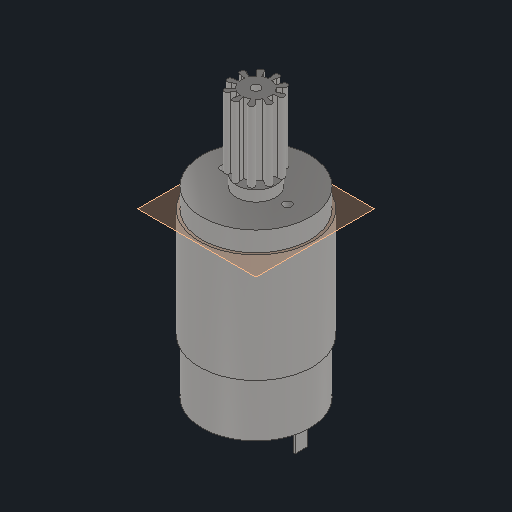
# Autodesk Inventor part: rs390
Saved by Autodesk Inventor 2023 (Build 270158000, 158)
## iProperties
Created: 2024-04-13
Part Number: rs390
Material: Steel, Mild
Document SubType Name: Modeling
Designer: szymo
Density: 7.85 g/cm^3
Appearance: Semi-Polished
Mass: 105 g
Surface Area: 71.7705 cm^2
Volume: 30.7913 cm^3
Author: szymo
Autodesk Inventor part; units mm, degrees
ref_plane "YZ Plane" through (0, 0, 0) normal (1, 0, 0) x (0, 1, 0)
ref_plane "XZ Plane" through (0, 0, 0) normal (0, 1, 0) x (-1, 0, 0)
ref_plane "XY Plane" through (0, 0, 0) normal (0, 0, 1) x (1, 0, 0)
sketch "Sketch1" plane through (0, 0, 0) normal (0, 1, 0) x (-1, 0, 0)
  circle A0 centre (0, 0) radius 13.7
  dimension "d0" = 27.4
  constraints: 1 centre point, 1 coincident
  measures "d0" diameter of A0
extrude "Extrusion1" add sketch "Sketch1" along normal blind 46.5
sketch "Sketch2" plane through (0, 46.5, 0) normal (0, 1, 0) x (1, 0, 0)
  circle A0 centre (0, 0) radius 13.7 projected
  circle A1 centre (0, 0) radius 5
  dimension "d3" = 10
  constraints: 1 centre point, 1 coincident
  measures "d3" diameter of A1
extrude "Extrusion2" add sketch "Sketch2" along normal blind 2.7 contours A1
sketch "Sketch3" plane through (0, 46.5, 0) normal (0, 1, 0) x (1, 0, 0)
  circle A0 centre (0, 0) radius 5 projected
  circle A1 centre (0, 0) radius 5 projected
  circle A2 centre (0, 0) radius 13.7 projected
  circle A3 centre (0, 0) radius 13.7 projected
  line L0 (-13.7, 0) -> (13.7, 0)
  point P0 (-8, 0)
  point P1 (8, 0)
  dimension "d6" = 16
  dimension "d7" = 5.7
  dimension "d8" = 5.7
  constraints: 2 end point, 2 point on circle, 2 point on line, 1 horizontal
  measures "d6" distance of point (-8, 0) point (8, 0)
  measures "d7" distance of L0.start point (-8, 0)
  measures "d8" distance of L0.end point (8, 0)
hole "Hole1" at (-8, 46.5, 0) at (8, 46.5, 0) direction (0, -1, 0) diameter 2.1129 depth 2.8 thread size "M2.6x0.45" class "6H" standard "ISO Metric profile"
ref_plane "Work Plane1" through (0, 41.5, 0) normal (0, 1, 0) x (1, 0, 0)
sketch "Sketch4" plane through (0, 41.5, 0) normal (0, 1, 0) x (1, 0, 0)
  circle A0 centre (0, 0) radius 14.375
  dimension "d17" = 28.75
  constraints: 1 centre point, 1 coincident
  measures "d17" diameter of A0
extrude "Extrusion3" add sketch "Sketch4" against normal blind 27.7
sketch "Sketch5" plane through (0, 0, 0) normal (0, -1, 0) x (1, 0, 0)
  circle A0 centre (0, 0) radius 5
  dimension "d20" = 10
  constraints: 1 centre point, 1 coincident
  measures "d20" diameter of A0
extrude "Extrusion4" add sketch "Sketch5" along normal blind 4
sketch "Sketch6" plane through (0, 0, 0) normal (0, -1, 0) x (1, 0, 0)
  circle A0 centre (0, 0) radius 5 projected
  circle A1 centre (0, 0) radius 5 projected
  circle A2 centre (0, 0) radius 13.7 projected
  circle A3 centre (0, 0) radius 13.7 projected
  line L0 (13.7, 0) -> (-13.7, 0)
  line L1 (-11.5, 1.5) -> (-12, 1.5)
  line L2 (-12, 1.5) -> (-12, -1.5)
  line L3 (-12, -1.5) -> (-11.5, -1.5)
  line L4 (-11.5, -1.5) -> (-11.5, 1.5)
  line L5 (11.5, 1.5) -> (11, 1.5)
  line L6 (11, 1.5) -> (11, -1.5)
  line L7 (11, -1.5) -> (11.5, -1.5)
  line L8 (11.5, -1.5) -> (11.5, 1.5)
  dimension "d23" = 22.5
  dimension "d24" = 0.5
  dimension "d25" = 0.5
  dimension "d26" = 11.5
  dimension "d27" = 11.5
  dimension "d28" = 3
  dimension "d29" = 3
  dimension "d30" = 1.5
  dimension "d31" = 1.5
  constraints: 18 end point, 4 horizontal, 4 parallel, 2 perpendicular, 2 point on circle, 2 point on line
  measures "d23" distance between parallel lines of L6 L4
  measures "d24" distance of L6.end L7.end
  measures "d25" distance between parallel lines of L4 L2
  measures "d26" distance from line of A2.centre L8
  measures "d27" distance from line of A0.centre L4
  measures "d28" distance between parallel lines of L3 L1
  measures "d29" distance of L7.end L5.start
  measures "d30" distance between parallel lines of L0 L7
  measures "d31" distance between parallel lines of L0 L5
extrude "Extrusion5" add sketch "Sketch6" along normal blind 6 contours L6 L5 L8 L0 | L0 L8 L7 L6 | L4 L3 L2 L0 | L0 L2 L1 L4
sketch "Sketch7" plane through (0, 49.2, 0) normal (0, 1, 0) x (1, 0, 0)
  circle A0 centre (0, 0) radius 1.1
  dimension "d34" = 2.2
  constraints: 1 centre point, 1 coincident
  measures "d34" diameter of A0
extrude "Extrusion6" add sketch "Sketch7" along normal blind 13.5
sketch "Sketch8" plane through (0, 62.7, 0) normal (0, 1, 0) x (1, 0, 0)
  circle A0 centre (0, 0) radius 1.1 projected
  circle A1 centre (0, 0) radius 5.925
  circle A2 centre (0, 0) radius 3.625
  circle A3 centre (0, 0) radius 4.775
  arc A4 (0.5843, 4.7391) -> (-0.5843, 4.7391) centre (0, 5.1881) ccw
  line L0 (0.4436, 3.5978) -> (0.725, 5.8805)
  line L1 (-0.4436, 3.5978) -> (-0.725, 5.8805)
  line L2 (-1.7559, 3.1714) -> (-2.8699, 5.1835)
  line L3 (-2.4736, 2.6499) -> (-4.043, 4.3313)
  arc A5 (-2.3129, 4.1775) -> (-3.2583, 3.4906) centre (-3.0495, 4.1973) ccw
  line L4 (-3.2846, 1.5336) -> (-5.3686, 2.5067)
  line L5 (-3.5587, 0.6899) -> (-5.8167, 1.1277)
  arc A6 (-4.3266, 2.0202) -> (-4.6877, 0.9088) centre (-4.9342, 1.6032) ccw
  line L6 (-3.5587, -0.6899) -> (-5.8167, -1.1277)
  line L7 (-3.2846, -1.5336) -> (-5.3686, -2.5067)
  arc A7 (-4.6877, -0.9088) -> (-4.3266, -2.0202) centre (-4.9342, -1.6032) ccw
  line L8 (-2.4736, -2.6499) -> (-4.043, -4.3313)
  line L9 (-1.7559, -3.1714) -> (-2.8699, -5.1835)
  arc A8 (-3.2583, -3.4906) -> (-2.3129, -4.1775) centre (-3.0495, -4.1973) ccw
  line L10 (-0.4436, -3.5978) -> (-0.725, -5.8805)
  line L11 (0.4436, -3.5978) -> (0.725, -5.8805)
  arc A9 (-0.5843, -4.7391) -> (0.5843, -4.7391) centre (0, -5.1881) ccw
  line L12 (1.7559, -3.1714) -> (2.8699, -5.1835)
  line L13 (2.4736, -2.6499) -> (4.043, -4.3313)
  arc A10 (2.3129, -4.1775) -> (3.2583, -3.4906) centre (3.0495, -4.1973) ccw
  line L14 (3.2846, -1.5336) -> (5.3686, -2.5067)
  line L15 (3.5587, -0.6899) -> (5.8167, -1.1277)
  arc A11 (4.3266, -2.0202) -> (4.6877, -0.9088) centre (4.9342, -1.6032) ccw
  line L16 (3.5587, 0.6899) -> (5.8167, 1.1277)
  line L17 (3.2846, 1.5336) -> (5.3686, 2.5067)
  arc A12 (4.6877, 0.9088) -> (4.3266, 2.0202) centre (4.9342, 1.6032) ccw
  line L18 (2.4736, 2.6499) -> (4.043, 4.3313)
  line L19 (1.7559, 3.1714) -> (2.8699, 5.1835)
  arc A13 (3.2583, 3.4906) -> (2.3129, 4.1775) centre (3.0495, 4.1973) ccw
  point P0 (3.7689, -4.0376)
  dimension "d37" = 11.85
  dimension "d38" = 7.25
  dimension "d39" = 1.45
  dimension "d43" = 1.15
  dimension "d44" = 1.15
  dimension "d47" = 360
  constraints: 40 end point, 26 point on circle, 20 midpoint, 13 centre point, 3 coincident, 101 other
  measures "d37" diameter of A1
  measures "d38" diameter of A2
  measures "d39" distance of L1.end L0.end
  measures "d43" radial gap between concentric circles of A3 A2
  measures "d44" radial gap between concentric circles of A1 A3
extrude "Extrusion7" add sketch "Sketch8" along normal blind 5.5 and the other way blind 12.5 contours A12 L16 A3 L17 | A12 L16 | A11 L14 A3 L15 | L15 A11 | L17 A12 | L16 A2 L17 A3 | A11 L14 | A3 L14 A2 L15 | A2 | A13 L18 A3 L19 | A13 L18 | L18 A2 L19 A3 | A10 L12 A3 L13 | L13 A10 | A3 L12 A2 L13 | L19 A13 | A10 L12 | L0 A2 L1 A3 | L0 A4 | A3 L1 A4 L0 | L11 A9 L10 A3 | A3 L10 A2 L11 | A9 L11 | A4 L1 | L10 A9 | L2 A2 L3 A3 | A3 L3 A5 L2 | L2 A5 | L9 A8 L8 A3 | A3 L8 A2 L9 | A8 L9 | A5 L3 | L8 A8 | L4 A2 L5 A3 | A3 L5 A6 L4 | L4 A6 | L7 A7 L6 A3 | A3 L6 A2 L7 | A7 L7 | A6 L5 | L6 A7
equation "\"d7\" = d8"
equation "\"d26\" = d27"
equation "\"d30\" = d31"
equation "\"d43\" = d44"
equation "\"d41\" = d42"
body "Solid1"
